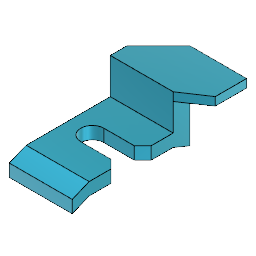
Endstop Flag X (Autodesk Fusion 360 design; units mm, degrees)
Autodesk Fusion 360 part; units mm, degrees
ref_plane "WorkPlane3" through (38.5, 10, 36) normal (1, 0, 0) x (0, 1, 0)
sketch "Sketch3" plane through (38.5, 64, 26) normal (1, 0, 0) x (0, 1, 0)
  line L0 (20, -10) -> (24, -10)
  line L1 (24, -10) -> (24, 8.3252)
  line L2 (24, 8.3252) -> (20, 10)
  line L3 (0, 10) -> (-4, 8.3252)
  line L4 (-4, 8.3252) -> (-4, -10)
  line L5 (-4, -10) -> (0, -10)
  line L6 (0, -10) -> (0, 6)
  line L7 (0, 6) -> (20, 6)
  line L8 (20, 6) -> (20, -10)
  line L9 (-4, 8.3252) -> (-4, 11.3252)
  line L10 (-4, 11.3252) -> (0, 13)
  line L11 (0, 13) -> (20, 13)
  line L12 (20, 13) -> (24, 11.3252)
  line L13 (24, 11.3252) -> (24, 8.3252)
  line L14 (10, 10) -> (10, 13) construction
  line L15 (20, 10) -> (0, 10)
  dimension "d6921" = 3
  dimension "d6928" = 3
extrude "Extrude1" add sketch "Sketch3" against normal blind 12 from surface at -2 contours L2 L3 L9 L10 L11 L12 L13 L15
sketch "Sketch4" plane through (36.5, 0, 0) normal (1, 0, 0) x (0, 1, 0)
  line L0 (84, 36) -> (88, 34.3252)
  line L1 (88, 34.3252) -> (88, 37.3252)
  line L2 (88, 37.3252) -> (84, 39)
  line L3 (84, 39) -> (64, 39)
  line L4 (64, 39) -> (60, 37.3252)
  line L5 (60, 37.3252) -> (60, 34.3252)
  line L6 (60, 34.3252) -> (64, 36)
  line L7 (64, 36) -> (84, 36)
  line L8 (88, 37.3252) -> (88, 45.5)
  line L9 (88, 45.5) -> (95.5, 45.5)
  line L10 (95.5, 45.5) -> (95.5, 47.5)
  line L11 (95.5, 47.5) -> (84, 47.5)
  line L12 (84, 47.5) -> (84, 39)
  line L13 (88, 45.5) -> (88, 47.5)
  dimension "d6930" = 8.5
  dimension "d6931" = 2
  dimension "d6937" = 7.5
extrude "Extrude2" add sketch "Sketch4" against normal blind 15
extrude "Extrude3" add sketch "Sketch4" along normal blind 6 contours L9 L10 L11 L13
sketch "Sketch5" plane through (0, 0, 39) normal (0, 0, 1) x (-1, 0, 0)
  line L0 (-36.5, -64) -> (-36.5, -84)
  line L1 (-36.5, -84) -> (-21.5, -84)
  line L2 (-21.5, -84) -> (-21.5, -64)
  line L3 (-21.5, -64) -> (-36.5, -64)
  line L4 (-36.5, -74) -> (-21.5, -74) construction
  circle A0 centre (-27.25, -74) radius 2.75
  line L5 (-27.25, -76.75) -> (-36.5, -76.75)
  line L6 (-36.5, -71.25) -> (-27.25, -71.25)
  dimension "d6939" = 5.5
  dimension "d6974" = 3
  measures "d6939" diameter of A0
extrude "Extrude4" cut sketch "Sketch5" against normal blind 12 contours L0 A0 L5 L6 | A0
chamfer "Chamfer3" distance 2 angle 45 2 edges at (36.5, 76.75, 37.5) (36.5, 71.25, 37.5)
chamfer "Chamfer4" distance 4 distance2 6 1 edges at (36.5, 88, 46.5) measured on face at (36.5, 86.6667, 39.6084)
chamfer "Chamfer5" distance 7.5 angle 45 1 edges at (21.5, 95.5, 46.5)
equation "d6928 = d6921"
named bodies: "X Endstop Flag V3"
